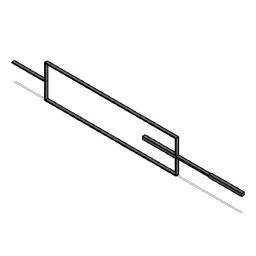
droplet (Autodesk Fusion 360 design; units mm, degrees)
Autodesk Fusion 360 part; units mm, degrees
sketch "Sketch1" plane through (0, 0, 0) normal (0, 0, 1) x (1, 0, 0)
  line L0 (0, 0.05) -> (5, 0.05)
  line L1 (5, 0.05) -> (5, -0.05) construction
  line L2 (5, -0.05) -> (0, -0.05)
  line L3 (0, -0.05) -> (0, 0.05)
  line L4 (5, 0.05) -> (5, 2.5)
  line L5 (5, 2.5) -> (25, 2.5)
  line L6 (25, 2.5) -> (25, 0.1)
  line L7 (25, 0.1) -> (30, 0.1)
  line L8 (30, -0.1) -> (25, -0.1)
  line L9 (25, -0.1) -> (25, -2.5)
  line L10 (25, -2.5) -> (5, -2.5)
  line L11 (5, -2.5) -> (5, -0.05)
  line L12 (30, 0.1) -> (30, 0.2)
  line L13 (19.9, 0.2) -> (19.9, -0.2)
  line L14 (30, -0.4037) -> (30, -0.1)
  line L15 (5.1, 2.4) -> (24.9, 2.4)
  line L16 (24.9, 2.4) -> (24.9, 0.2)
  line L17 (24.9, 0.2) -> (19.9, 0.2)
  line L18 (19.9, 0.2) -> (19.9, -0.2)
  line L19 (19.9, -0.2) -> (24.9, -0.2)
  line L20 (24.9, -0.2) -> (24.9, -2.4)
  line L21 (24.9, -2.4) -> (5.1, -2.4)
  line L22 (5.1, -2.4) -> (5.1, 2.4)
  line L23 (24.9, 0.2) -> (19.9, 0.2)
  line L24 (25, 0.2) -> (24.9, 0.2) construction
  line L25 (19.9, -0.2) -> (24.9, -0.2)
  line L26 (24.9, -0.2) -> (25, -0.6007) construction
  line L27 (30, -0.1) -> (30, -0.2)
  line L28 (30, -0.2) -> (35, -0.2)
  line L29 (35, -0.2) -> (35, 0.2)
  line L30 (35, 0.2) -> (30, 0.2)
  line L31 (30, 0.2) -> (30, 0.1)
  point P0 (19.9, 0)
  point P1 (35, 0)
  dimension "d56" = 0.1
  dimension "d57" = 5
  dimension "d58" = 0.2
  dimension "d59" = 5
  dimension "d60" = 5
  dimension "d64" = 0.1
  dimension "d65" = 0.1
  dimension "d66" = 0.1
  dimension "d67" = 0.1
  dimension "d68" = 0.4
  dimension "d70" = 0.2
  dimension "d71" = 5
  dimension "d72" = 20
  dimension "d73" = 5
  dimension "d74" = 0.1
  dimension "d76" = 5
  dimension "d77" = 0.4
  dimension "d78" = 0.2
  dimension "spacer" = 5
  dimension "d80" = 0.1
  dimension "d81" = 2.5
  constraint horizontal L0
  constraint vertical L1
  constraint horizontal L2
  constraint vertical L3
  constraint midpoint origin L3
  constraint perpendicular L0 L4
  constraint perpendicular L4 L5
  constraint perpendicular L0 L6
  constraint perpendicular L6 L7
  constraint perpendicular L8 L9
  constraint perpendicular L9 L10
  constraint perpendicular L7 L12
  constraint perpendicular L7 L13
  constraint perpendicular L8 L14
  constraint horizontal L25
  constraint collinear L6 L9
  constraint perpendicular L4 L15
  constraint perpendicular L15 L16
  constraint perpendicular L16 L17
  constraint perpendicular L17 L18
  constraint perpendicular L18 L19
  constraint perpendicular L17 L20
  constraint perpendicular L11 L21
  constraint vertical L22
  constraint coincident L6 L24.start
  constraint coincident L9 L26.end
  constraint horizontal L23
  constraint perpendicular L8 L27
  constraint perpendicular L27 L28
  constraint perpendicular L28 L29
  constraint perpendicular L27 L30
  constraint perpendicular L7 L31
  constraint midpoint L13 P0
  constraint midpoint L29 P1
  measures "d56" distance of L0 L2
  measures "d57" distance of L0.start L0.end
  measures "d58" distance of L7 L8
  measures "d59" distance of L6.end L7.end
  measures "d60" distance of L8.start L8.end
  measures "d64" distance of L6 L16
  measures "d65" distance of L4 L22
  measures "d66" distance of L5 L15
  measures "d67" distance of L10 L21
  measures "d68" distance of L17 L19
  measures "d70" distance of origin L17
  measures "d71" distance of L18 L19.end
  measures "d72" distance of L4.end L5.end
  measures "d73" distance of L5 L10
  measures "d74" distance of L9 L20
  measures "d76" distance of L13.end L19.end
  measures "d77" distance of L28 L30
  measures "d78" distance of origin L30
  measures "spacer" distance of L27.end L28.end
  measures "d80" distance of origin L7
  measures "d81" distance of origin L10
extrude "Extrude2" add sketch "Sketch1" along normal blind 0.4
equation "d1000 = channelwidth"
equation "d11 = d1000 * 2.2"
equation "d1001 = depth"
equation "mouth_user = 0.1 mm" comment "User entered value."
equation "mouth_size = d1000 + 0.5 mm" comment "Multiplier to user entered value"
equation "channelwidth = 0.1 mm"
equation "depth = 0.4 mm"
equation "length = 20 mm"
equation "neckwidth = 0.2 mm"
equation "inputwidth = neckwidth * 2"
equation "outletwidth = inputwidth"
equation "necklength = 5 mm"
equation "d56 = channelwidth"
equation "d57 = spacer"
equation "d58 = neckwidth"
equation "d59 = necklength"
equation "d60 = necklength"
equation "d64 = channelwidth"
equation "d65 = channelwidth"
equation "d66 = channelwidth"
equation "d67 = channelwidth"
equation "d68 = inputwidth"
equation "d70 = inputwidth / 2"
equation "d71 = inputlength"
equation "d72 = length"
equation "d74 = channelwidth"
equation "d76 = inputlength"
equation "d77 = outletwidth"
equation "d78 = outletwidth / 2"
equation "d80 = neckwidth / 2"
equation "d81 = d73 / 2"
equation "inputlength = 5 mm"
